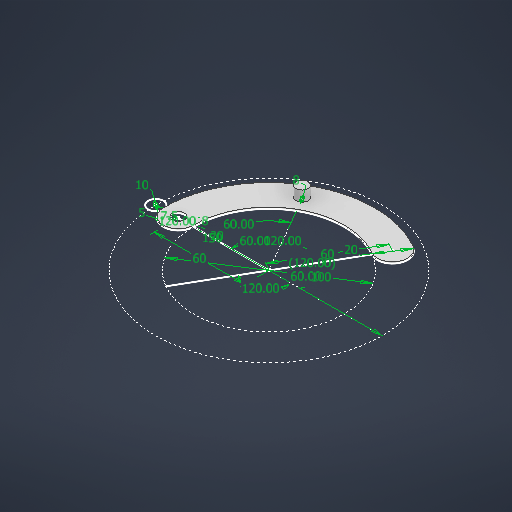
# Autodesk Inventor part: Part15
Saved by Autodesk Inventor 2026.2 (Build 302298000, 298)
## iProperties
Created: 2025-12-30
Part Number: Part15
Material: Generic
Document SubType Name: Modeling
Designer: Cobble
Density: 1 g/cm^3
Appearance: Default
Author: Cobble
Autodesk Inventor part; units mm, degrees
ref_plane "YZ Plane" through (0, 0, 0) normal (1, 0, 0) x (0, 1, 0)
ref_plane "XZ Plane" through (0, 0, 0) normal (0, 1, 0) x (-1, 0, 0)
ref_plane "XY Plane" through (0, 0, 0) normal (0, 0, 1) x (1, 0, 0)
sketch "Sketch1" plane through (0, 0, 0) normal (0, 0, 1) x (1, 0, 0)
  circle A0 centre (0, 0) radius 50 construction
  line L0 (0, 0) -> (-60, 0)
  circle A1 centre (-60, 0) radius 10
  line L1 (0, 0) -> (-23.6561, 40.9735) construction
  line L2 (0, 0) -> (-50, 0) construction
  line L3 (0, 0) -> (-25, -43.3013)
  line L4 (0, 0) -> (50, 0) construction
  line L5 (0, 0) -> (65, 0) construction
  line L6 (0, 0) -> (30, 51.9615)
  line L7 (0, 0) -> (60, 0) construction
  circle A2 centre (30, 51.9615) radius 10
  arc A3 (35, 60.6218) -> (-70, 0) centre (0, 0) ccw
  arc A4 (25, 43.3013) -> (-50, 0) centre (0, 0) ccw
  line L8 (0, 0) -> (25, 43.3013) construction
  line L9 (0, 0) -> (-50, 0) construction
  line L10 (-60, 0) -> (-63.75, -6.4952)
  line L11 (-60, 0) -> (-52.5, 0) construction
  circle A5 centre (-60, 0) radius 4
  circle A6 centre (-63.75, -6.4952) radius 2.5
  circle A7 centre (0, 0) radius 75 construction
  line L12 (0, 0) -> (-75, 0) construction
  circle A8 centre (-75, 0) radius 5
  line L13 (-25, 43.3013) -> (-35, 60.6218)
  line L14 (0, 0) -> (70, 0) construction
  circle A9 centre (-30, 51.9615) radius 4
  point P0 (25, 43.3013)
  point P1 (-62, -3.4641)
  point P2 (-56, 0)
  dimension "d14" = 20
  dimension "d23" = 150
  dimension "d0" = 100
  dimension "d1" = 60
  dimension "d2" = 20
  dimension "d3" = 60
  dimension "d4" = 120
  dimension "d12" = 60
  dimension "d13" = 60
  dimension "d15" = 120
  dimension "d19" = 7.5
  dimension "d20" = 120
  dimension "d21" = 8
  dimension "d22" = 5
  dimension "d24" = 10
  dimension "d25" = 120
  dimension "d26" = 60
  dimension "d27" = 8
  constraints: 30 end point, 11 coincident, 8 centre point, 8 point on circle, 6 horizontal, 3 equal length, 3 point on line, 1 horizontal alignment, 1 midpoint, 5 other
  measures "d0" diameter of A0
  measures "d1" distance of L0.start L0.end
  measures "d2" diameter of A1
  measures "d3" angle of L1 L2
  measures "d4" angle of L3 L4
  measures "d12" distance of L1.start L6.end
  measures "d13" angle of L7 L6
  measures "d15" angle of L8 L9
  measures "d19" distance of L10.start L10.end
  measures "d20" angle of L10 L11
  measures "d21" diameter of A5
  measures "d22" diameter of A6
  measures "d24" diameter of A8
  measures "d25" angle of L14 L13
  measures "d26" angle of L2 L13
  measures "d27" diameter of A9
extrude "Extrusion1" add sketch "Sketch1" along normal blind 1 contours A1 A6 L10 A5 L0 | L0 A5 L10 A6 A1 | A1 A3 L13 A9 A4 | A4 L13 A9 A3 A2 | A2 | A6 | A9 L13 | L13 A9
extrude "Extrusion2" add sketch "Sketch1" along normal blind 8 contours A9 L13 | L13 A9
body "Solid1"
